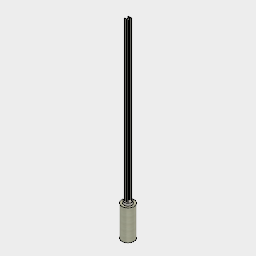
Support (Autodesk Fusion 360 design; units mm, degrees)
Autodesk Fusion 360 part; units mm, degrees
sketch "Sketch1" plane through (0, 0, 0) normal (0, 1, 0) x (1, 0, 0)
  line L0 (0, 0) -> (100, 0) construction
  line L1 (100, 0) -> (100, 190) construction
  line L2 (100, 190) -> (-100, 190) construction
  line L3 (-100, 190) -> (-100, 0) construction
  line L4 (-100, 0) -> (0, 0) construction
  line L5 (-100, 10) -> (-100, 0)
  line L6 (-100, 0) -> (100, 0)
  line L7 (100, 10) -> (100, 0)
  line L8 (100, 190) -> (100, 180)
  line L9 (100, 190) -> (-100, 190)
  line L10 (-100, 190) -> (-100, 180)
  line L11 (0, 190) -> (0, 0) construction
  line L12 (-3.25, 162) -> (-3.25, 28)
  line L13 (3.25, 162) -> (3.25, 28)
  line L14 (-100, 10) -> (-21.25, 10)
  line L15 (21.25, 10) -> (100, 10)
  line L16 (-100, 180) -> (-21.25, 180)
  line L17 (21.25, 180) -> (100, 180)
  arc A0 (-3.25, 162) -> (-21.25, 180) centre (-21.25, 162) ccw
  arc A1 (21.25, 180) -> (3.25, 162) centre (21.25, 162) ccw
  arc A2 (3.25, 28) -> (21.25, 10) centre (21.25, 28) ccw
  arc A3 (-21.25, 10) -> (-3.25, 28) centre (-21.25, 28) ccw
  dimension "d7" = 100
  dimension "d8" = 190
  dimension "d9" = 200
  dimension "d10" = 190
  dimension "d12" = 10
  dimension "d13" = 10
  dimension "d14" = 3.25
  dimension "d15" = 3.25
  dimension "d16" = 18
  measures "d7" distance of L0.start L0.end
  measures "d8" distance of L0.end L1.end
  measures "d9" distance of L1.end L2.end
  measures "d10" distance of L2.end L3.end
  measures "d12" distance of L2 L16
  measures "d13" distance of L4 L14
  measures "d14" distance of L11 L12
  measures "d15" distance of L11 L13
  measures "d16" radius of A0
extrude "Extrude1" add sketch "Sketch1" along normal blind 7250 and the other way blind 2250 makes body 1
ref_plane "WorkPlane1" through (0, -950, 0) normal (0, 1, 0) x (0, 0, 1)
ref_plane "WorkPlane2" through (0, -2500, 0) normal (0, 1, 0) x (0, 0, 1)
sketch "Sketch2" plane through (0, -950, 0) normal (0, 1, 0) x (1, 0, 0)
  line L0 (0, 0) -> (0, 95)
  circle A0 centre (0, 95) radius 310
  dimension "d23" = 95
  dimension "d24" = 620
  measures "d23" distance of L0.start L0.end
  measures "d24" diameter of A0
extrude "Extrude2" add sketch "Sketch2" against normal blind 1550 separate body makes body 2
sketch "Sketch4" plane through (0, 0, 0) normal (1, 0, 0) x (0, 0, -1)
  line L0 (95, -950) -> (-105, -950)
  line L1 (-105, -950) -> (-105, -830) construction
  line L2 (95, -950) -> (95, -830) construction
  line L3 (95, -830) -> (-105, -830) construction
  line L4 (95, -830) -> (-90, -830)
  line L5 (-90, -830) -> (-105, -950)
  line L6 (95, -830) -> (95, -950)
  point P0 (95, -950)
  dimension "d28" = 200
  dimension "d29" = 120
  dimension "d30" = 120
  dimension "d31" = 185
  measures "d28" distance of P0 L0.end
  measures "d29" distance of L0.end L1.end
  measures "d30" distance of P0 L2.end
  measures "d31" distance of L2.end L4.end
revolve "Revolve1" add sketch "Sketch4" angle 360 about axis through (0, -830, -95) along (0, -1, 0) separate body makes body 3
sketch "Sketch de construction - Positionnement piquetage" plane through (0, 0, 0) normal (0, 1, 0) x (1, 0, 0)
  circle A0 centre (0, 95) radius 310 construction
  line L0 (0, 0) -> (0, 95) construction
  line L1 (0, 0) -> (-295.0847, 0) construction
  line L2 (0, 0) -> (295.0847, 0) construction
equation "d14 = ( 6.5 / 2 ) * 1 mm"
named bodies: "HEA200", "Mast"
